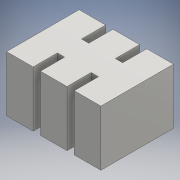
# Autodesk Inventor part: CommonGNDVDD
Saved by Autodesk Inventor 2016 (Build 200138000, 138)
## iProperties
Created: 2016-05-02
Part Number: CommonGNDVDD
Material: ABS Plastic
Document SubType Name: Modeling
Designer: Artur
Density: 1.06 g/cm^3
Appearance: Smooth - White
Author: Artur
Autodesk Inventor part; units mm, degrees
ref_plane "YZ Plane" through (0, 0, 0) normal (1, 0, 0) x (0, 1, 0)
ref_plane "XZ Plane" through (0, 0, 0) normal (0, 1, 0) x (-1, 0, 0)
ref_plane "XY Plane" through (0, 0, 0) normal (0, 0, 1) x (1, 0, 0)
sketch "Sketch1" plane through (0, 0, 0) normal (0, 0, 1) x (1, 0, 0)
  line L0 (0, 3.6903) -> (0, -33.2554)
  line L1 (0, 0) -> (5.5, 0)
  line L2 (5.5, 0) -> (5.5, -10)
  line L3 (5.5, -10) -> (8.5, -10)
  line L4 (8.5, -10) -> (8.5, 0)
  line L5 (8.5, 0) -> (19.5, 0)
  line L6 (19.5, 0) -> (19.5, -30)
  line L7 (19.5, -30) -> (8.5, -30)
  line L8 (8.5, -30) -> (8.5, -20)
  line L9 (8.5, -20) -> (5.5, -20)
  line L10 (5.5, -20) -> (5.5, -30)
  line L11 (0, -30) -> (5.5, -30)
  line L12 (0, 0) -> (-5.5, 0)
  line L13 (-5.5, 0) -> (-5.5, -10)
  line L14 (-5.5, -10) -> (-8.5, -10)
  line L15 (-8.5, -10) -> (-8.5, 0)
  line L16 (-8.5, 0) -> (-19.5, 0)
  line L17 (-19.5, 0) -> (-19.5, -30)
  line L18 (-19.5, -30) -> (-8.5, -30)
  line L19 (-8.5, -30) -> (-8.5, -20)
  line L20 (-8.5, -20) -> (-5.5, -20)
  line L21 (-5.5, -20) -> (-5.5, -30)
  line L22 (0, -30) -> (-5.5, -30)
  dimension "d0" = 5.5
  dimension "d1" = 10
  dimension "d2" = 3
  dimension "d3" = 11
  dimension "d4" = 30
  dimension "d5" = 11
  dimension "d6" = 10
  dimension "d7" = 5.5
  dimension "d8" = 3
  constraints: 46 end point, 10 symmetric about line, 9 point on line, 8 perpendicular, 2 horizontal, 1 coincident, 1 vertical
  measures "d0" distance of L1.start L1.end
  measures "d1" distance of L1.end L2.end
  measures "d2" distance of L2.end L3.end
  measures "d3" distance of L4.end L5.end
  measures "d4" distance of L5.end L6.end
  measures "d5" distance of L6.end L7.end
  measures "d6" distance of L7.end L8.end
  measures "d7" distance of L11.start L10.end
  measures "d8" distance of L8.end L9.end
extrude "Extrusion1" add sketch "Sketch1" along normal blind 23
equation "\"d5\" = d3"
equation "\"d6\" = d1"
equation "\"d7\" = d0"
equation "\"d8\" = d2"
body "Solid1"
